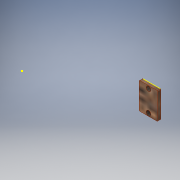
# Autodesk Inventor part: termo
Saved by Autodesk Inventor 2019.5 (Build 235369000, 369)
## iProperties
Created: 2022-10-11
Part Number: termo
Material: Wood (Oak)
Document SubType Name: Modeling
Designer: ASUS
Density: 0.76 g/cm^3
Appearance: White Oak - Natural Medium Gloss
Author: ASUS
Autodesk Inventor part; units mm, degrees
ref_plane "YZ Plane" through (0, 0, 0) normal (1, 0, 0) x (0, 1, 0)
ref_plane "XZ Plane" through (0, 0, 0) normal (0, 1, 0) x (-1, 0, 0)
ref_plane "XY Plane" through (0, 0, 0) normal (0, 0, 1) x (1, 0, 0)
sketch "Sketch1" plane through (0, 0, 0) normal (0, 0, 1) x (1, 0, 0)
  line L0 (77.1826, 34.3167) -> (88.1826, 34.3167)
  line L1 (88.6826, 33.8167) -> (88.6826, 17.8167)
  line L2 (88.1826, 17.3167) -> (77.1826, 17.3167)
  line L3 (76.6826, 17.8167) -> (76.6826, 33.8167)
  arc A0 (77.1826, 34.3167) -> (76.6826, 33.8167) centre (77.1826, 33.8167) ccw
  arc A1 (88.6826, 33.8167) -> (88.1826, 34.3167) centre (88.1826, 33.8167) ccw
  arc A2 (88.1826, 17.3167) -> (88.6826, 17.8167) centre (88.1826, 17.8167) ccw
  arc A3 (76.6826, 17.8167) -> (77.1826, 17.3167) centre (77.1826, 17.8167) ccw
  line L4 (82.4065, 34.3167) -> (82.6826, 17.3167)
  point P0 (0, 0)
  point P1 (88.6826, 17.3167)
  point P2 (88.6826, 34.3167)
  point P3 (76.6826, 17.3167)
  dimension "d0" = 12
  dimension "d1" = 17
  dimension "d2" = 0.5
  constraints: 10 end point, 8 point on circle, 8 tangent, 7 point on line, 4 centre point, 3 equal radius, 2 parallel, 1 horizontal, 1 midpoint, 1 perpendicular
  measures "d0" distance of point (88.683, 17.317) point (76.683, 17.317)
  measures "d1" distance of point (88.683, 34.317) point (88.683, 17.317)
  measures "d2" radius of A0
extrude "Extrusion1" add sketch "Sketch1" along normal blind 2
sketch "Sketch2" plane through (0, 0, 2) normal (0, 0, 1) x (1, 0, 0)
  point P0 (0, 0)
  point P1 (82.7526, 32.5302)
hole "Hole1" at (82.7526, 32.5302, 2) direction (0, 0, -1) diameter 3 depth 55.5
sketch "Sketch3" plane through (0, 0, 2) normal (0, 0, 1) x (1, 0, 0)
  point P0 (0, 0)
  point P1 (82.7236, 19.0448)
hole "Hole2" at (82.7236, 19.0448, 2) direction (0, 0, -1) diameter 3 depth 55.5
sketch "Sketch5" plane through (0, 0, 0) normal (0, 0, 1) x (1, 0, 0)
  line L0 (88.1826, 34.3167) -> (77.1826, 34.3167) projected
  line L1 (77.1826, 17.3167) -> (88.1826, 17.3167) projected
  line L2 (83.824, 30.7891) -> (81.5769, 30.7891) construction
  line L3 (81.5769, 30.7891) -> (81.5769, 20.7942) construction
  line L4 (81.5769, 20.7942) -> (83.824, 20.7942) construction
  line L5 (83.824, 20.7942) -> (83.824, 30.7891) construction
  point P0 (0, 0)
  constraints: 2 other
body "Solid1"
